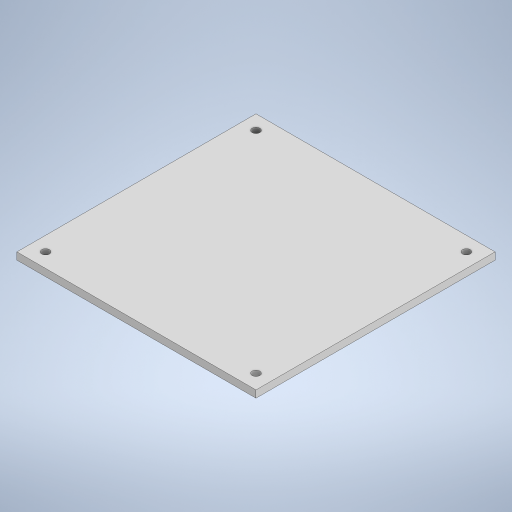
# Autodesk Inventor part: TopPlate
Saved by Autodesk Inventor 2023 (Build 270158000, 158)
## iProperties
Created: 2022-07-23
Part Number: TopPlate
Material: Generic
Document SubType Name: Modeling
Designer: Aditya Bansal
Density: 1 g/cm^3
Appearance: Default
Author: Aditya Bansal
Autodesk Inventor part; units mm, degrees
ref_plane "YZ Plane" through (0, 0, 0) normal (1, 0, 0) x (0, 1, 0)
ref_plane "XZ Plane" through (0, 0, 0) normal (0, 1, 0) x (-1, 0, 0)
ref_plane "XY Plane" through (0, 0, 0) normal (0, 0, 1) x (1, 0, 0)
sketch "Sketch1" plane through (0, 0, 0) normal (0, 1, 0) x (-1, 0, 0)
  line L0 (0, 0) -> (100, 0)
  line L1 (100, 0) -> (100, -100)
  line L2 (100, -100) -> (0, -100)
  line L3 (0, -100) -> (0, 0)
  line L4 (100, 0) -> (97, 0) construction
  line L5 (97, 0) -> (97, -100) construction
  line L6 (97, -100) -> (100, -100) construction
  line L7 (100, -100) -> (100, 0) construction
  line L8 (97, 0) -> (3, 0) construction
  line L9 (3, 0) -> (3, -3) construction
  line L10 (3, -3) -> (97, -3) construction
  line L11 (97, -3) -> (97, 0) construction
  line L12 (3, 0) -> (0, 0) construction
  line L13 (0, 0) -> (0, -100) construction
  line L14 (0, -100) -> (3, -100) construction
  line L15 (3, -100) -> (3, 0) construction
  line L16 (3, -100) -> (97, -100) construction
  line L17 (97, -100) -> (97, -97) construction
  line L18 (97, -97) -> (3, -97) construction
  line L19 (3, -97) -> (3, -100) construction
  line L20 (97, -3) -> (91, -3) construction
  line L21 (91, -3) -> (91, -9) construction
  line L22 (91, -9) -> (97, -9) construction
  line L23 (97, -9) -> (97, -3) construction
  line L24 (97, -97) -> (91, -97) construction
  line L25 (91, -97) -> (91, -91) construction
  line L26 (91, -91) -> (97, -91) construction
  line L27 (97, -91) -> (97, -97) construction
  line L28 (3, -3) -> (9, -3) construction
  line L29 (9, -3) -> (9, -9) construction
  line L30 (9, -9) -> (3, -9) construction
  line L31 (3, -9) -> (3, -3) construction
  line L32 (3, -97) -> (9, -97) construction
  line L33 (9, -97) -> (9, -91) construction
  line L34 (9, -91) -> (3, -91) construction
  line L35 (3, -91) -> (3, -97) construction
  circle A0 centre (94, -6) radius 1.6
  circle A1 centre (94, -94) radius 1.6
  circle A2 centre (6, -6) radius 1.6
  circle A3 centre (6, -94) radius 1.6
  point P0 (91, -6)
  point P1 (94, -9)
  point P2 (9, -6)
  point P3 (6, -9)
  point P4 (91, -94)
  point P5 (94, -91)
  dimension "d0" = 100
  dimension "d2" = 3
  dimension "d3" = 6
  dimension "d4" = 3.2
  constraints: 72 end point, 18 parallel, 11 equal length, 9 horizontal, 9 perpendicular, 6 midpoint, 4 centre point, 4 horizontal alignment, 4 vertical alignment, 3 equal radius, 2 point on line
  measures "d0" distance of L1.end L2.end
  measures "d2" distance between parallel lines of L0 L10
  measures "d3" distance of L20.end L21.end
  measures "d4" diameter of A0
extrude "Extrusion1" add sketch "Sketch1" along normal blind 3
body "Solid1"
